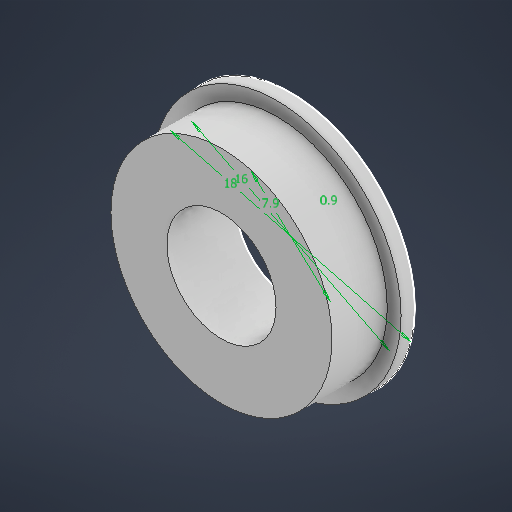
# Autodesk Inventor part: 16mmOD Belt Bearing Half
Saved by Autodesk Inventor 2025.1 (Build 291241000, 241)
## iProperties
Created: 2024-11-11
Part Number: 16mmOD Belt Bearing Half
Material: Generic
Document SubType Name: Modeling
Designer: jerem
Density: 1 g/cm^3
Appearance: Default
Author: jerem
Autodesk Inventor part; units mm, degrees
ref_plane "YZ Plane" through (0, 0, 0) normal (1, 0, 0) x (0, 1, 0)
ref_plane "XZ Plane" through (0, 0, 0) normal (0, 1, 0) x (-1, 0, 0)
ref_plane "XY Plane" through (0, 0, 0) normal (0, 0, 1) x (1, 0, 0)
sketch "Sketch1" plane through (0, 0, 0) normal (0, 0, 1) x (1, 0, 0)
  circle A0 centre (0, 0) radius 3.95
  circle A1 centre (0, 0) radius 8
  circle A2 centre (0, 0) radius 9
  circle A3 centre (0, 0) radius 4.85
  dimension "d0" = 7.9
  dimension "d1" = 16
  dimension "d2" = 18
  dimension "d7" = 0.9
  constraints: 4 centre point, 4 coincident
  measures "d0" diameter of A0
  measures "d1" diameter of A1
  measures "d2" diameter of A2
  measures "d7" radial gap between concentric circles of A3 A0
extrude "Extrusion1" add sketch "Sketch1" along normal blind 1 contours A2
extrude "Extrusion2" add sketch "Sketch1" along normal blind 5 contours A1 | A3
body "Solid1"
